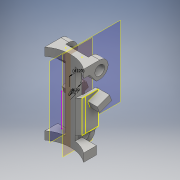
# Autodesk Inventor part: back_pack_8
Saved by Autodesk Inventor 2016 (Build 200138000, 138)
## iProperties
Created: 2016-06-06
Part Number: back_pack_8
Material: Generic
Document SubType Name: Modeling
Designer: ajar021
Density: 1 g/cm^3
Appearance: Default
Author: ajar021
Autodesk Inventor part; units mm, degrees
ref_plane "YZ Plane" through (0, 0, 0) normal (1, 0, 0) x (0, 1, 0)
ref_plane "XZ Plane" through (0, 0, 0) normal (0, 1, 0) x (-1, 0, 0)
sketch "Sketch1" plane through (0, 0, 0) normal (0, 0, 1) x (1, 0, 0)
  line L0 (-6, 1) -> (6, 1)
  line L1 (6, 1) -> (6, -1)
  line L2 (6, -1) -> (-6, -1)
  line L3 (-6, -1) -> (-6, 1)
  line L4 (-6, 1) -> (6, -1) construction
  line L5 (6, 1) -> (-6, -1) construction
  line L6 (-6, -1) -> (-6, -3)
  line L7 (6, -1) -> (6, -3)
  arc A0 (6, -3) -> (-6, -3) centre (0, -11) ccw
  point P0 (0, 0)
  dimension "d0" = 12
  dimension "d1" = 2
  dimension "d2" = 2
  dimension "d3" = 2
  constraints: 16 end point, 2 midpoint, 2 parallel, 2 point on circle, 2 vertical, 1 centre point, 1 horizontal, 1 perpendicular
  measures "d0" distance of L0.start L0.end
  measures "d1" distance of L0.end L1.end
  measures "d2" distance of L2.end L6.end
  measures "d3" distance of L1.end L7.end
extrude "Extrusion1" add sketch "Sketch1" against normal blind 25
sketch "Sketch2" plane through (-6, 1, 0) normal (0, 1, 0) x (1, 0, 0)
  line L0 (12, 0) -> (12, 25) projected
  line L1 (0, 0) -> (0, 25) projected
  line L2 (0, 0) -> (0, 2.5)
  line L3 (12, 0) -> (12, 2.5)
  line L4 (0, 25) -> (0, 22.5)
  line L5 (12, 25) -> (12, 22.5)
  line L6 (0, 2.5) -> (4.5, 2.5)
  line L7 (4.5, 2.5) -> (4.5, 22.5)
  line L8 (4.5, 22.5) -> (0, 22.5)
  line L9 (0, 22.5) -> (0, 2.5)
  line L10 (12, 2.5) -> (7.5, 2.5)
  line L11 (7.5, 2.5) -> (7.5, 22.5)
  line L12 (7.5, 22.5) -> (12, 22.5)
  line L13 (12, 22.5) -> (12, 2.5)
  point P0 (6, 0)
  dimension "d6" = 2.5
  dimension "d7" = 2.5
  dimension "d8" = 2.5
  dimension "d9" = 2.5
  dimension "d10" = 12
  dimension "d11" = 4.5
  dimension "d12" = 4.5
  constraints: 24 end point, 4 parallel, 4 point on line, 2 horizontal, 2 perpendicular
  measures "d6" distance of L1.start L2.end
  measures "d7" distance of L1.end L4.end
  measures "d8" distance of L0.end L5.end
  measures "d9" distance of L0.start L3.end
  measures "d10" distance of L0.start L1.start
  measures "d11" distance of L8.end L7.end
  measures "d12" distance of L11.end L12.end
extrude "Extrusion2" cut sketch "Sketch2" against normal blind 25
sketch "Sketch3" plane through (-6, 1, 0) normal (0, 1, 0) x (1, 0, 0)
  line L0 (7.5, 2.5) -> (7.5, 22.5) projected
  line L1 (4.5, 22.5) -> (4.5, 2.5) projected
  line L2 (0, 0) -> (0, 2.5) projected
  line L3 (4.5, 2.5) -> (4.5, 3.5)
  line L4 (7.5, 2.5) -> (7.5, 3.5)
  line L5 (4.5, 3.5) -> (4.5, 5)
  line L6 (4.5, 5) -> (5, 5)
  line L7 (5, 5) -> (5, 3.5)
  line L8 (5, 3.5) -> (4.5, 3.5)
  line L9 (7.5, 3.5) -> (7.5, 5)
  line L10 (7.5, 5) -> (7, 5)
  line L11 (7, 5) -> (7, 3.5)
  line L12 (7, 3.5) -> (7.5, 3.5)
  line L13 (4.5, 2.5) -> (4.5, 7)
  line L14 (4.5, 7) -> (0, 7)
  line L15 (0, 7) -> (0, 8.5)
  line L16 (0, 8.5) -> (4.5, 8.5)
  line L17 (7.5, 7) -> (12, 7)
  line L18 (12, 7) -> (12, 8.5)
  line L19 (12, 8.5) -> (7.5, 8.5)
  line L20 (4.5, 7) -> (4.5, 21)
  line L21 (7.5, 7) -> (7.5, 21)
  line L22 (4.5, 21) -> (7.5, 21)
  line L23 (7.5, 21) -> (7.5, 22.5)
  line L24 (7.5, 22.5) -> (4.5, 22.5)
  line L25 (4.5, 22.5) -> (4.5, 21)
  line L26 (4.5, 21) -> (3.5, 21)
  line L27 (3.5, 21) -> (3.5, 11)
  line L28 (3.5, 11) -> (4.5, 11)
  line L29 (4.5, 11) -> (4.5, 21)
  line L30 (7.5, 21) -> (8.5, 21)
  line L31 (8.5, 21) -> (8.5, 11)
  line L32 (8.5, 11) -> (7.5, 11)
  line L33 (7.5, 11) -> (7.5, 21)
  line L34 (3.5, 21) -> (4.5, 22.5)
  line L35 (7.5, 22.5) -> (8.5, 21)
  line L36 (7.5, 5) -> (8, 5)
  line L37 (8, 5) -> (8, 3.5)
  line L38 (8, 3.5) -> (7.5, 3.5)
  line L39 (4.5, 5) -> (4, 5)
  line L40 (4, 5) -> (4, 3.5)
  line L41 (4, 3.5) -> (5, 3.5)
  point P0 (12, 25)
  point P1 (12, 0)
  point P2 (6, 0)
  dimension "d15" = 1
  dimension "d16" = 1.5
  dimension "d17" = 0.5
  dimension "d18" = 0.5
  dimension "d19" = 4.5
  dimension "d20" = 1.5
  dimension "d21" = 14
  dimension "d22" = 4.5
  dimension "d23" = 4.5
  dimension "d24" = 14
  dimension "d25" = 25
  dimension "d26" = 1.5
  dimension "d29" = 1
  dimension "d30" = 10
  dimension "d31" = 1
  dimension "d34" = 0.5
  dimension "d35" = 0.5
  dimension "d50" = 10
  constraints: 78 end point, 20 point on line, 15 perpendicular, 7 parallel, 3 horizontal, 1 collinear
  measures "d15" distance of L1.end L3.end
  measures "d16" distance of L3.end L5.end
  measures "d17" distance of L5.end L6.end
  measures "d18" distance of L9.end L10.end
  measures "d19" distance of L1.end L13.end
  measures "d20" distance of L14.end L15.end
  measures "d21" distance of L13.end L20.end
  measures "d22" distance of L18.end L19.end
  measures "d23" distance of L15.end L16.end
  measures "d24" distance from line of L21.end L17
  measures "d25" distance of point (12, 25) point (12, 0)
  measures "d26" distance of L22.end L23.end
  measures "d29" distance of L28.end L27.end
  measures "d30" distance of L26.end L27.end
  measures "d31" distance of L31.end L32.end
  measures "d34" distance of L9.end L36.end
  measures "d35" distance of L5.end L39.end
  measures "d50" distance of L30.end L31.end
extrude "Extrusion3" add sketch "Sketch3" along normal blind 4 contours L0 L30 L31 L32 | L22 L1 L24 L0 | L0 L35 L30 | L26 L34 L1 | L1 L28 L27 L26
ref_plane "Work Plane1" through (-1.5, 1, -12.5) normal (-1, 0, 0) x (0, 0, 1)
sketch "Sketch8" plane through (-2.5, -1.3175, -11) normal (-1, 0, 0) x (0, 0, 1)
  line L0 (-10, 6.3175) -> (-11.5, 6.3175) projected
  line L1 (0, 0) -> (-10, 0) projected
  line L2 (0, 2.3175) -> (0, 6.3175) projected
  line L3 (-10, 6.3175) -> (0, 6.3175) projected
  line L4 (-10, 2.3175) -> (0, 2.3175) projected
  line L5 (-1.7443, 2.0961) -> (-3.6237, 2.7802)
  line L6 (-0.3763, 5.8549) -> (-2.2557, 6.5389)
  line L7 (0, 2.3175) -> (-10, 2.3175) projected
  line L8 (0, 2.3175) -> (-10, 2.3175) projected
  line L9 (-1.7443, 2.0961) -> (-0.3763, 5.8549)
  line L10 (-2.2557, 6.5389) -> (-3.6237, 2.7802)
  point P0 (11, 1.3175)
  point P1 (-2, 4.3175)
  dimension "d119" = 4
  dimension "d120" = 4
  dimension "d127" = 2
  constraints: 8 end point
  measures "d119" distance of L5.start L6.start
  measures "d120" distance between parallel lines of L3 L4
  measures "d127" distance of L5.end L5.start
sketch "Sketch9" plane through (2.5, -1.3175, -21) normal (1, 0, 0) x (0, 0, -1)
  line L0 (0, 2.3175) -> (0, 6.3175) projected
  line L1 (0, 0) -> (-10, 0) projected
  line L2 (-6.3763, 2.7802) -> (-8.2557, 2.0961)
  line L3 (-10, 6.3175) -> (0, 6.3175) projected
  line L4 (-10, 6.3175) -> (0, 6.3175) projected
  line L5 (0, 6.3175) -> (-10, 6.3175) projected
  line L6 (-10, 6.3175) -> (-9, 6.3175)
  line L7 (-7, 2.3175) -> (-7, 6.3175) projected
  line L8 (-10, 2.3175) -> (0, 2.3175) projected
  line L9 (-8, 5.3175) -> (-8, 2.3175)
  line L10 (-6.3763, 3.7802) -> (-8.2557, 3.0961)
  line L11 (-8.2557, 3.0961) -> (-9.6237, 6.8549)
  line L12 (-9.6237, 6.8549) -> (-7.7443, 7.5389)
  line L13 (-7.7443, 7.5389) -> (-6.3763, 3.7802)
  line L14 (-9, 7.3175) -> (-7, 3.3175) construction
  line L15 (-7, 7.3175) -> (-9, 3.3175) construction
  point P0 (-21, 1.3175)
  point P1 (-9, 2.3175)
  point P2 (-9, 1.1588)
  dimension "d133" = 3
  dimension "d134" = 2
  dimension "d135" = 4
  dimension "lean_angle" = 20
  constraints: 18 end point, 2 midpoint, 2 parallel, 2 perpendicular, 2 point on line, 1 collinear
  measures "d133" distance of L9.start L9.end
  measures "d134" distance of L11.end L12.end
  measures "d135" distance of L12.end L10.start
  measures "lean_angle" angle of L11 L9
ref_plane "Work Plane33" through (-1.5, 5, -11) normal (-1, 0, 0) x (0, 0, -1)
sketch "Sketch12" plane through (-1.5, 5, -11) normal (-1, 0, 0) x (0, 0, -1)
  line L0 (11.5, 4) -> (11.5, 0) projected
  line L1 (14, 8) -> (14, 4) projected
  line L2 (14, 4) -> (11.5, 0)
  line L3 (11.5, 4) -> (14, 4) projected
  line L4 (14, 0) -> (11.5, 0)
  line L5 (11.5, 0) -> (13.6217, 0) construction
  line L6 (13.6217, 0) -> (14.1176, 2) construction
  line L7 (14.1176, 2) -> (14, 4) construction
  spline S0 degree 3 poles (11.5, 0) (13.6217, 0) (14.1176, 2) (14, 4) knots 1 1 1 1 2 2 2 2
  point P0 (-11, 5)
  constraints: 4 end point, 1 horizontal, 4 other
extrude "Extrusion12" add sketch "Sketch12" against normal up to surface (3 mm away)
sketch "Sketch15" plane through (2.5, -1.3175, -21) normal (1, 0, 0) x (0, 0, -1)
  line L0 (1.5, 2.3175) -> (4, 2.3175) projected
  line L1 (1.5, 2.3175) -> (1.5, 6.3175) projected
  line L2 (4, 2.3175) -> (1.5, 2.3175) projected
  line L3 (1.5, 2.3175) -> (1.5, 3.3175)
  circle A0 centre (1.5, 3.3175) radius 1.3
  point P0 (-21, 1.3175)
  dimension "d77" = 1
  dimension "d78" = 2.6
  constraints: 2 end point, 1 centre point, 1 coincident, 1 point on line, 1 other
  measures "d77" distance of L3.start L3.end
  measures "d78" diameter of A0
extrude "Extrusion14" cut sketch "Sketch15" against normal up to surface (12 mm away) from surface at 3.5
sketch "Sketch16" plane through (-6, 5, 0) normal (0, 1, 0) x (1, 0, 0)
  line L0 (3.5, 11) -> (4.5, 11) projected
  line L1 (4.5, 11) -> (4.5, 21) projected
  line L2 (7.5, 21) -> (7.5, 11) projected
  line L3 (7.5, 11) -> (8.5, 11) projected
  line L4 (4.5, 11) -> (4.3, 11)
  line L5 (4.3, 11) -> (4.3, 21)
  line L6 (4.3, 21) -> (4.5, 21)
  line L7 (7.5, 11) -> (7.5, 21) projected
  line L8 (7.5, 11) -> (7.7, 11)
  line L9 (7.7, 11) -> (7.7, 21)
  line L10 (7.7, 21) -> (7.5, 21)
  line L11 (7.5, 21) -> (7.5, 11)
  point P0 (6, 0)
  dimension "d81" = 0.2
  dimension "d82" = 0.2
  dimension "d83" = 0.2
  constraints: 14 end point, 2 equal length, 2 perpendicular, 2 point on line
  measures "d81" distance of L0.end L4.end
  measures "d82" distance of L5.end L1.end
  measures "d83" distance of L2.end L8.end
extrude "Extrusion15" cut sketch "Sketch16" against normal up to surface (4 mm away)
sketch "Sketch20" plane through (6, -3, 0) normal (1, 0, 0) x (0, 0, -1)
  line L0 (0, 4) -> (2.5, 4) projected
  line L1 (0, 4) -> (4.5, 4)
  line L2 (0, 4) -> (0, 5) projected
  line L3 (0, 4) -> (0, 5)
  line L4 (22.5, 1.8869) -> (2.5, 1.8869) projected
  line L5 (2.5, 1.8869) -> (22.5, 1.8869) projected
  line L6 (21, 4) -> (2.5, 4) projected
  line L7 (2.5, 1.8869) -> (2.5, 4)
  line L8 (0, 4) -> (5.2, 4)
  line L9 (2.5, 4) -> (21, 4) projected
  line L10 (5.2, 4) -> (5.2, 5)
  line L11 (5.2, 5) -> (0, 5) construction
  arc A0 (5.2, 5) -> (0, 5) centre (2.6, 5) ccw
  line L12 (2.5, 1.8869) -> (5.2, 4)
  dimension "d130" = 5.2
  dimension "d131" = 2.6
  constraints: 14 end point, 3 perpendicular, 2 point on circle, 2 point on line, 1 centre point, 1 collinear, 1 horizontal, 1 midpoint
  measures "d130" distance of L0.start L8.end
  measures "d131" radius of A0
extrude "Extrusion18" add sketch "Sketch20" against normal blind 2.5
sketch "Sketch24" plane through (-6, 1, 0) normal (0, -1, 0) x (1, 0, 0)
  line L0 (4.3, -21) -> (4.3, -11) projected
  line L1 (3.5, -11) -> (4.3, -11) projected
  line L2 (3.5, -21) -> (3.5, -11) projected
  line L3 (3.9462, -21.6693) -> (3.5, -21) projected
  line L4 (3.9462, -21.6693) -> (4.5, -21.6693) projected
  line L5 (4.5, -21.6693) -> (4.5, -21) projected
  line L6 (4.5, -21) -> (4.3, -21) projected
  line L7 (7.5, -22.5) -> (7.5, -2.5) projected
  line L8 (7.7, -21) -> (7.5, -21) projected
  line L9 (7.5, -21) -> (7.5, -21.6693) projected
  line L10 (7.5, -21.6693) -> (8.0538, -21.6693) projected
  line L11 (8.5, -21) -> (8.0538, -21.6693) projected
  line L12 (8.5, -11) -> (8.5, -21) projected
  line L13 (7.7, -11) -> (8.5, -11) projected
  line L14 (7.7, -11) -> (7.7, -21) projected
  line L15 (0, -23.3307) -> (4.5, -23.3307) projected
  line L16 (0, -22.5) -> (0, -23.3307) projected
  line L17 (4.5, -22.5) -> (0, -22.5) projected
  line L18 (4.5, -21.6693) -> (4.5, -22.5) projected
  line L19 (3.9462, -21.6693) -> (4.5, -21.6693) projected
  line L20 (4.5, -22.5) -> (3.9462, -21.6693) projected
  line L21 (8.0538, -21.6693) -> (7.5, -22.5) projected
  line L22 (7.5, -21.6693) -> (8.0538, -21.6693) projected
  line L23 (7.5, -22.5) -> (7.5, -21.6693) projected
  line L24 (12, -22.5) -> (7.5, -22.5) projected
  line L25 (12, -23.3307) -> (12, -22.5) projected
  line L26 (7.5, -2.5) -> (12, -2.5) projected
  line L27 (12, 0) -> (12, -2.5) projected
  line L28 (0, 0) -> (12, 0) projected
  line L29 (0, 0) -> (0, -2.5) projected
  line L30 (0, -2.5) -> (4.5, -2.5) projected
  line L31 (4.5, -2.5) -> (4.5, -22.5) projected
  line L32 (4.5, -22.5) -> (0, -22.5) projected
  line L33 (0, -22.5) -> (0, -25) projected
  line L34 (12, -25) -> (0, -25) projected
  line L35 (12, -22.5) -> (12, -25) projected
  line L36 (12, -22.5) -> (7.5, -22.5) projected
  line L37 (7.5, -22.5) -> (7.5, -2.5) projected
  line L38 (7.5, -2.5) -> (12, -2.5) projected
  line L39 (12, 0) -> (12, -2.5) projected
  line L40 (0, 0) -> (12, 0) projected
  line L41 (0, 0) -> (0, -2.5) projected
  line L42 (0, -2.5) -> (4.5, -2.5) projected
  line L43 (4.5, -2.5) -> (4.5, -22.5) projected
  line L44 (4.5, -22.5) -> (0, -22.5) projected
  line L45 (0, -22.5) -> (0, -25) projected
  line L46 (12, -25) -> (0, -25) projected
  line L47 (12, -22.5) -> (12, -25) projected
  line L48 (12, -22.5) -> (7.5, -22.5) projected
  line L49 (7.5, -22.5) -> (7.5, -2.5) projected
  line L50 (4.5, -30) -> (4.5, 5) projected
  line L51 (8.5, -11) -> (7.5, -11)
  line L52 (7.5, -2.5) -> (7.5, -21) projected
  line L53 (7.5, -22.5) -> (4.5, -22.5) projected
  line L54 (7.5, -11) -> (7.5, -22.5)
  line L55 (8.3667, -21.2) -> (7.5, -22.5) projected
  line L56 (7.5, -22.5) -> (8.5, -21)
  line L57 (8.5, -11) -> (8.5, -21) projected
  line L58 (8.5, -11) -> (8.5, -21) projected
  line L59 (8.5, -11) -> (8.5, -21)
  line L60 (7.5, -11) -> (7.5, -22.5)
  line L61 (3.5, -21) -> (3.5, -11) projected
  line L62 (3.5, -11) -> (3.5, -21)
  line L63 (3.5, -21) -> (3.5, -11) projected
  line L64 (3.5, -21) -> (4.5, -22.5)
  line L65 (3.5, -11) -> (4.5, -11)
  line L66 (3.5, -21) -> (4.5, -22.5)
  line L67 (4.5, -22.5) -> (4.5, -11)
  line L68 (4.5, -2.5) -> (4.5, -22.5) projected
  line L69 (4.5, -11) -> (4.5, -22.5)
  line L70 (4.5, -23.3307) -> (4.5, -22.5) projected
  line L71 (7.5, -23.3307) -> (12, -23.3307) projected
  line L72 (7.5, -22.5) -> (7.5, -23.3307) projected
  point P0 (6, 0)
  point P1 (3.5, -12)
  point P2 (3.5, -14)
  point P3 (8.5, -14)
  point P4 (8.5, -12)
  constraints: 22 end point, 3 collinear, 3 point on line, 3 vertical, 1 perpendicular, 5 other
extrude "Extrusion22" add sketch "Sketch24" along normal blind 1
extrude "Extrusion23" add sketch "Sketch9" along normal blind 3 contours L13 L7 L10 L11 L3 | L3 L11 L12 L13 | L13 L10 L7
ref_plane "Work Plane34" through (0, 5, -11) normal (1, 0, 0) x (0, 0, -1)
sketch "Sketch22" plane through (6, -3, 0) normal (1, 0, 0) x (0, 0, -1)
  line L0 (0.3944, 5) -> (5.1266, 5) construction
  circle A0 centre (2.7605, 5) radius 1.5
  point P0 (0, 3)
  dimension "d132" = 3
  constraints: 2 end point, 1 centre point, 1 coincident, 1 horizontal, 1 midpoint
  measures "d132" diameter of A0
extrude "Extrusion20" cut sketch "Sketch22" against normal through all
sketch "Sketch25" plane through (2.5, -1.3175, -21) normal (-1, 0, 0) x (0, 0, 1)
  line L0 (9.4281, 6.3175) -> (7.2998, 6.3175) projected
  line L1 (9.4281, 6.3175) -> (9.6237, 6.8549) projected
  line L2 (9.6237, 6.8549) -> (7.7443, 7.5389) projected
  line L3 (7.7443, 7.5389) -> (7.2998, 6.3175) projected
  point P0 (21, 1.3175)
extrude "Extrusion25" add sketch "Sketch25" along normal up to surface (0.8 mm away)
sketch "Sketch26" plane through (1.5, 1, -11) normal (0, 0, 1) x (1, 0, 0)
  line L0 (0, -1) -> (1, -1)
  line L1 (1, -1) -> (0, -2.1131)
  line L2 (0, -2.1131) -> (0, -1)
  point P0 (-1.5, -1)
  constraints: 6 end point, 1 horizontal, 1 vertical
extrude "Extrusion26" add sketch "Sketch26" against normal up to surface (10 mm away)
mirror "Mirror2" about plane through (0, 5, -11) normal (1, 0, 0) of "Extrusion18", "Extrusion23", "Extrusion20", "Extrusion25", "Extrusion26"
sketch "Sketch27" plane through (2.5, 5, -13.7002) normal (1, 0, 0) x (0, 0, -1)
  line L0 (-0.9559, -3.2214) -> (-2.1284, 0) projected
  line L1 (-2.7002, 0) -> (-2.1284, 0) projected
  line L2 (-2.7002, -5) -> (-2.7002, 0) projected
  line L3 (7.2998, -5) -> (-2.7002, -5) projected
  line L4 (7.2998, -5) -> (7.2998, 0) projected
  line L5 (0, 0) -> (7.2998, 0) projected
  line L6 (0, 0) -> (0.9235, -2.5374) projected
  line L7 (0.9235, -2.5374) -> (-0.9559, -3.2214) projected
  line L8 (7.2998, -4) -> (-2.7002, -4) projected
  line L9 (-8.5002, -4) -> (-11.2002, -6.1131) projected
  point P0 (-13.7002, -5)
equation "\"d7\" = d6"
equation "\"d8\" = d6"
equation "\"d9\" = d6"
equation "\"d12\" = d11"
equation "\"d18\" = d17"
equation "\"d22\" = d23"
equation "\"d24\" = d21"
equation "\"d31\" = d29"
equation "\"d34\" = d17"
equation "\"d50\" = d30"
equation "\"d82\" = d81"
body "Solid1"
